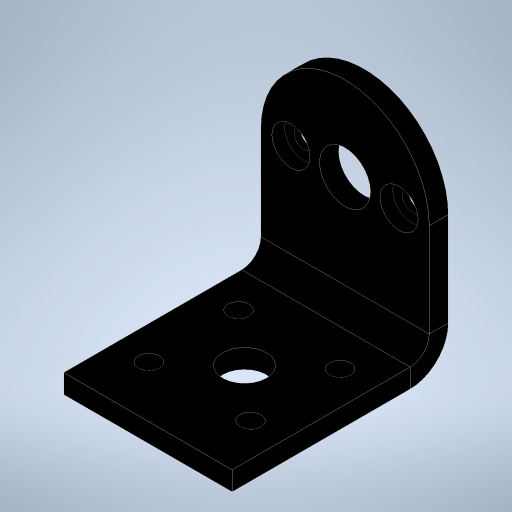
# Autodesk Inventor part: JGA25-370-bracket
Saved by Autodesk Inventor 2023 (Build 270158000, 158)
## iProperties
Created: 2022-05-10
Part Number: JGA25-370-bracket
Material: Aluminum 6061
Document SubType Name: Sheet Metal
Designer: Dan
Density: 2.7 g/cm^3
Sheet Metal Rule: Default_mm
Appearance: Anodized - Black
Author: Dan
Autodesk Inventor part; units mm, degrees
ref_plane "YZ Plane" through (0, 0, 0) normal (1, 0, 0) x (0, 1, 0)
ref_plane "XZ Plane" through (0, 0, 0) normal (0, 1, 0) x (-1, 0, 0)
ref_plane "XY Plane" through (0, 0, 0) normal (0, 0, 1) x (1, 0, 0)
sketch "Sketch4" plane through (0, 0, 0) normal (0, 0, 1) x (1, 0, 0)
  line L0 (0, 0) -> (26.5, 0)
  line L1 (26.5, 0) -> (26.5, 20.75)
  line L2 (0, 20.75) -> (0, 0)
  arc A0 (26.5, 20.75) -> (0, 20.75) centre (13.25, 20.75) ccw
  line L3 (-1.1061, 34) -> (25.3939, 34) construction
  dimension "d70" = 26.5
  dimension "d71" = 34
  measures "d70" distance of L0.start L0.end
  measures "d71" distance between parallel lines of L3 L0
extrude "Plate3" add sketch "Sketch4" along normal blind 3
sketch "Sketch5" plane through (26.5, 3, 0) normal (0, -1, 0) x (1, 0, 0)
  line L0 (-26.5, 0) -> (0, 0)
  line L1 (0, 0) -> (0, 34)
  line L2 (0, 34) -> (-26.5, 34)
  line L3 (-26.5, 34) -> (-26.5, 0)
  constraints: 6 end point, 1 horizontal, 1 perpendicular, 1 vertical
edge flange "Flange2" height 34 angle 90 thickness 3 bend radius 3 thickness toward (0, -1, 0) relief straight relief width 3 relief depth 1.5 edges at (13.25, 0, 3) wall of the first edge with corners at (0, 3, 0) (26.5, 3, 0) (26.5, 3, 34) (0, 3, 34)
bend "Bend2"
corner "Corner2"
sketch "Sketch8" plane through (0, 3, 3) normal (0, 0, 1) x (1, 0, 0)
  line L0 (26.5, 3) -> (0, 3) projected
  line L1 (13.25, 3) -> (13.25, 35.5458) construction
  line L2 (0, -3) -> (26.5, -3) projected
  point P0 (13.25, 17.75)
  point P1 (13.25, -3)
  dimension "d72" = 20.75
  constraints: 2 end point, 2 midpoint, 1 point on line, 1 vertical
  measures "d72" distance of point (13.25, -3) point (13.25, 17.75)
hole "Hole3" at (13.25, 20.75, 3) direction (0, 0, -1) diameter 8 end through all
sketch "Sketch9" plane through (0, 3, 3) normal (0, 0, 1) x (1, 0, 0)
  circle A0 centre (13.25, 17.75) radius 8.5 construction
  circle A1 centre (13.25, 17.75) radius 4 projected
  point P0 (0, -3)
  point P1 (4.75, 17.75)
  point P2 (21.75, 17.75)
  dimension "d69" = 17
  constraints: 2 horizontal alignment, 2 point on circle, 1 centre point, 1 coincident, 1 concentric
  measures "d69" distance of A0.end A0.start
hole "Hole4" at (4.75, 20.75, 3) at (21.75, 20.75, 3) direction (0, 0, -1) diameter 3 end through all counterbore diameter 6 counterbore depth 2
sketch "Sketch11" plane through (0, 3, 34) normal (0, 1, 0) x (1, 0, 0)
  line L0 (0, 0) -> (26.5, 0) projected
  line L1 (13.25, 0) -> (13.25, 41.3955) construction
  point P0 (0, 34)
  point P1 (13.25, 15.2)
  dimension "d81" = 15.2
  constraints: 2 end point, 1 midpoint, 1 point on line, 1 vertical
  measures "d81" distance from line of L0 point (13.25, 15.2)
hole "Hole5" at (13.25, 3, 18.8) direction (0, -1, 0) diameter 6.9 end through all
sketch "Sketch12" plane through (0, 3, 34) normal (0, 1, 0) x (1, 0, 0)
  circle A0 centre (13.25, 15.2) radius 3.45 projected
  circle A1 centre (13.25, 15.2) radius 10.6631 construction
  line L0 (0, 0) -> (26.5, 0) projected
  point P0 (0, 34)
  point P1 (21.25, 8.15)
  point P2 (5.25, 8.15)
  point P3 (5.25, 22.25)
  point P4 (21.25, 22.25)
  dimension "d89" = 16
  dimension "d90" = 8.15
  constraints: 4 point on circle, 2 horizontal alignment, 1 centre point, 1 coincident, 1 vertical alignment
  measures "d89" distance of point (5.25, 8.15) point (21.25, 8.15)
  measures "d90" distance from line of L0 point (21.25, 8.15)
hole "Hole6" at (21.25, 3, 25.85) at (5.25, 3, 25.85) at (5.25, 3, 11.75) at (21.25, 3, 11.75) direction (0, -1, 0) diameter 3.3 end through all
equation "\"d27\" = Thickness"
equation "\"d28\" = BendReliefWidth"
equation "\"d29\" = BendReliefDepth"
equation "\"d30\" = MinimumRemnant"
equation "\"d31\" = TransitionRadius"
equation "\"d34\" = BendRadius"
equation "\"d35\" = CornerReliefSize"
equation "\"d36\" = GapSize"
equation "\"d37\" = JacobiRadiusSize"
equation "\"BendRadius\" = Thickness"
equation "\"BendReliefWidth\" = Thickness"
equation "\"BendReliefDepth\" = 0.5 * Thickness"
equation "\"CornerReliefSize\" = 4 * Thickness"
equation "\"MinimumRemnant\" = 2 * Thickness"
equation "\"TransitionRadius\" = BendRadius"
equation "\"JacobiRadiusSize\" = BendRadius"
equation "\"GapSize\" = Thickness"
equation "\"Thickness\" = 3"
body "Solid2"
